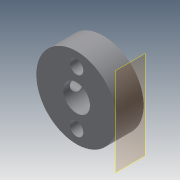
# Autodesk Inventor part: gearSupport
Saved by Autodesk Inventor 2015 (Build 190159000, 159)
## iProperties
Created: 2014-08-31
Part Number: gearSupport
Material: Generic
Document SubType Name: Modeling
Designer: shohei
Density: 1 g/cm^3
Appearance: Default
Author: shohei
Autodesk Inventor part; units mm, degrees
ref_plane "XZ Plane" through (0, 0, 0) normal (0, 1, 0) x (-1, 0, 0)
ref_plane "XY Plane" through (0, 0, 0) normal (0, 0, 1) x (1, 0, 0)
sketch "Sketch1" plane through (0, 0, 0) normal (0, 1, 0) x (-1, 0, 0)
  circle A0 centre (0, 0) radius 15
  circle A1 centre (0, 0) radius 5
  dimension "d0" = 30
  dimension "d1" = 10
  constraints: 2 centre point, 2 coincident
  measures "d0" diameter of A0
  measures "d1" diameter of A1
extrude "Extrusion1" add sketch "Sketch1" along normal blind 10
ref_plane "Work Plane1" through (15, 0, 0) normal (1, 0, 0) x (0, 1, 0)
sketch "Sketch2" plane through (0, 0, 0) normal (1, 0, 0) x (0, 1, 0)
  line L0 (-2, 0) -> (12, 0) projected
  line L1 (0, -21) -> (0, 21) projected
  circle A0 centre (5, 0) radius 2.5
  point P0 (0, 0)
  dimension "d5" = 5
  dimension "d6" = 5
  constraints: 1 centre point, 1 midpoint
  measures "d5" diameter of A0
  measures "d6" distance from line of L1 A0.centre
extrude "Extrusion2" cut sketch "Sketch2" against normal through all
sketch "Sketch3" plane through (0, 0, 0) normal (0, -1, 0) x (1, 0, 0)
  circle A0 centre (0, 0) radius 5 projected
  circle A1 centre (0, 0) radius 15 projected
  line L0 (-21.002, 0) -> (21.0003, 0) projected
  line L1 (0, -21) -> (0, 21) projected
  circle A2 centre (0, 10) radius 2.5
  circle A3 centre (0, -10) radius 2.5
  dimension "d10" = 5
  dimension "d11" = 10
  constraints: 2 centre point, 1 point on line, 1 symmetric about line, 1 other
  measures "d10" diameter of A2
  measures "d11" distance from line of L0 A2.centre
extrude "Extrusion3" cut sketch "Sketch3" against normal through all contours A2 L1 | L1 A2 | A3 L1 | L1 A3
equation "\"d4\" = 0.5 * d0"
body "Solid1"
